Autodesk Fusion 360 part; units mm, degrees
note: some values were not read from the file. Set by a fixed rule: which sketch regions a step uses.
(part 3 of 3)
  line L492 (149.0613, -85.0954) -> (151.4924, -71.3081)
  line L493 (151.4924, -71.3081) -> (165.2797, -73.7391)
  line L494 (165.2797, -73.7391) -> (162.8486, -87.5265)
  line L495 (162.8486, -87.5265) -> (149.0613, -85.0954)
  line L496 (155.3557, -130.0209) -> (152.9246, -143.8082)
  line L497 (152.9246, -143.8082) -> (139.1373, -141.3771)
  line L498 (139.1373, -141.3771) -> (141.5684, -127.5898)
  line L499 (141.5684, -127.5898) -> (155.3557, -130.0209)
  line L500 (139.9031, -107.9523) -> (137.472, -121.7396)
  line L501 (137.472, -121.7396) -> (123.6847, -119.3086)
  line L502 (123.6847, -119.3086) -> (126.1158, -105.5212)
  line L503 (126.1158, -105.5212) -> (139.9031, -107.9523)
  line L504 (158.6637, -111.2603) -> (156.2326, -125.0476)
  line L505 (156.2326, -125.0476) -> (142.4453, -122.6166)
  line L506 (142.4453, -122.6166) -> (144.8764, -108.8292)
  line L507 (144.8764, -108.8292) -> (158.6637, -111.2603)
  line L508 (129.4238, -86.7607) -> (143.2111, -89.1917)
  line L509 (143.2111, -89.1917) -> (140.78, -102.979)
  line L510 (140.78, -102.979) -> (126.9927, -100.548)
  line L511 (126.9927, -100.548) -> (129.4238, -86.7607)
  line L512 (166.1566, -68.7659) -> (152.3693, -66.3348)
  line L513 (152.3693, -66.3348) -> (154.8004, -52.5475)
  line L514 (154.8004, -52.5475) -> (168.5877, -54.9786)
  line L515 (168.5877, -54.9786) -> (166.1566, -68.7659)
  line L516 (107.7824, -70.7088) -> (105.3513, -84.4961)
  line L517 (105.3513, -84.4961) -> (91.564, -82.065)
  line L518 (91.564, -82.065) -> (93.9951, -68.2777)
  line L519 (93.9951, -68.2777) -> (107.7824, -70.7088)
  line L520 (130.2851, -52.7942) -> (127.854, -66.5815)
  line L521 (127.854, -66.5815) -> (114.0667, -64.1504)
  line L522 (114.0667, -64.1504) -> (116.4978, -50.3631)
  line L523 (116.4978, -50.3631) -> (130.2851, -52.7942)
  line L524 (157.0019, -158.2608) -> (176.1466, -49.6857)
  line L525 (176.1466, -49.6857) -> (132.1996, -41.9367)
  arc A0 (56.1359, -6.4676) -> (132.1996, -41.9367) centre (160.3539, 117.7346) ccw
  arc A1 (-132.1996, -41.9367) -> (-56.1359, -6.4676) centre (-160.3539, 117.7346) ccw
  line L526 (-132.1996, -41.9367) -> (-176.1466, -49.6857)
  line L527 (-176.1466, -49.6857) -> (-157.0019, -158.2608)
  line L528 (-157.0019, -158.2608) -> (-24.2252, -134.8487)
  arc A2 (24.2252, -134.8487) -> (-24.2252, -134.8487) centre (0, -272.2365) ccw
  line L529 (24.2252, -134.8487) -> (157.0019, -158.2608)
  line L530 (154.5684, -154.7854) -> (24.7461, -131.8943)
  line L531 (154.5684, -154.7854) -> (172.6712, -52.1192)
  line L532 (172.6712, -52.1192) -> (131.6786, -44.8911)
  line L533 (24.2252, -134.8487) -> (24.7461, -131.8943) construction
  line L534 (132.1996, -41.9367) -> (131.6786, -44.8911) construction
  arc A3 (54.2075, -8.7658) -> (131.6786, -44.8911) centre (160.3539, 117.7346) ccw
  line L535 (0, -2.5) -> (0, -20)
  arc A4 (-131.6786, -44.8911) -> (-54.2075, -8.7658) centre (-160.3539, 117.7346) ccw
  line L536 (-172.6712, -52.1192) -> (-131.6786, -44.8911)
  line L537 (-154.5684, -154.7854) -> (-172.6712, -52.1192)
  line L538 (-154.5684, -154.7854) -> (-24.7461, -131.8943)
  arc A5 (24.7461, -131.8943) -> (-24.7461, -131.8943) centre (0, -272.2365) ccw
  arc A6 (56.1359, -6.4676) -> (38.3662, 0) centre (38.3662, -27.6446) ccw
  line L539 (38.3662, 0) -> (-38.3662, 0)
  arc A7 (-38.3662, 0) -> (-56.1359, -6.4676) centre (-38.3662, -27.6446) ccw
  line L540 (38.3662, -3) -> (-38.3662, -3)
  line L541 (-38.3662, -3) -> (-38.3662, 0) construction
  line L542 (38.3662, -3) -> (38.3662, 0) construction
  arc A8 (54.2075, -8.7658) -> (38.3662, -3) centre (38.3662, -27.6446) ccw
  arc A9 (-38.3662, -3) -> (-54.2075, -8.7658) centre (-38.3662, -27.6446) ccw
  point P0 (54.2075, -8.7658)
  dimension "d428" = 3
  dimension "d429" = 3
  dimension "d430" = 3
  dimension "d431" = 3
  dimension "d436" = 3
  constraint perpendicular L47 L530
  constraint perpendicular L530 L531
  constraint perpendicular L524 L532
  constraint coincident A2.start L529.start
  constraint perpendicular L530 L533
  constraint coincident L525.end A0.end
  constraint perpendicular L532 L534
  constraint coincident L250 P0
  constraint coincident P0 A3.start
  constraint tangent L532 A3
  constraint symmetric L530.start L535 L537.start
  constraint symmetric L530.end L535 L538.end
  constraint symmetric L531.end L535 L536.start
  constraint symmetric L532.end L535 A4.start
  constraint symmetric P0 L535 A4.end
  constraint symmetric A3 L535 A4
  constraint tangent L530 A5
  constraint tangent L538 A5
  constraint horizontal L540
  constraint coincident L539.end A7.start
  constraint coincident A6.end L539.start
  constraint perpendicular L540 L542
  constraint perpendicular L540 L541
  constraint tangent L540 A8
  constraint tangent A4 A9
  measures "d428" distance of L524 L531
  measures "d429" distance of L529 L530
  measures "d430" distance of L525 L532
  measures "d431" distance of A0.start P0
  measures "d436" distance of L539 L540
extrude "Extrusion11" add sketch "Skizze4" along normal up to surface contours L524 L525 A0 A1 L526 L527 L528 A2 L529 A6 L539 A7 end surface through (0, 80, 16.8816) normal (0, 0.043619, -0.999048) offset 0 bodies 1
fillet "Abrundung1" radius 2 12 edges at (166.5742, 103.9733, 0) (154.1731, 45.8112, 0) (91.8329, 29.2091, 0) (47.8213, 1.6672, 0) (0, 0, 0) (-47.8213, 1.6672, 0) (-91.8329, 29.2091, 0) (-154.1731, 45.8112, 0) (-166.5742, 103.9733, 0) (-90.6135, 146.5547, 0) (0, 132.7292, 0) (90.6135, 146.5547, 0) on bodies 1
ref_plane "Arbeitsebene2" through (0, 0, 11) normal (0, 0, 1) x (1, 0, 0)
sketch "Skizze6" plane through (0, 0, 11) normal (0, 0, 1) x (1, 0, 0)
  line L0 (-153.7572, 153.627) -> (-24.9198, 130.9094)
  line L1 (-154.5684, 154.7854) -> (-24.7461, 131.8943)
  line L2 (-24.9198, 130.9094) -> (-24.7461, 131.8943) construction
  line L3 (-153.7572, 153.627) -> (-171.5128, 52.9304)
  line L4 (-172.6712, 52.1192) -> (-154.5684, 154.7854)
  line L5 (-171.5128, 52.9304) -> (-131.505, 45.8759)
  line L6 (-131.6786, 44.8911) -> (-172.6712, 52.1192)
  line L7 (-131.505, 45.8759) -> (-131.6786, 44.8911) construction
  line L8 (-38.3662, 4) -> (38.3662, 4)
  line L9 (38.3662, 3) -> (-38.3662, 3)
  line L10 (38.3662, 3) -> (38.3662, 4) construction
  line L11 (-38.3662, 4) -> (-38.3662, 3) construction
  arc A0 (-53.5647, 9.5318) -> (-131.505, 45.8759) centre (-160.3539, -117.7346) ccw
  arc A1 (-53.5647, 9.5318) -> (-38.3662, 4) centre (-38.3662, 27.6446) ccw
  arc A2 (-54.2075, 8.7658) -> (-131.6786, 44.8911) centre (-160.3539, -117.7346) ccw
  arc A3 (-54.2075, 8.7658) -> (-38.3662, 3) centre (-38.3662, 27.6446) ccw
  line L12 (0, 1.75) -> (0, 22.5)
  arc A4 (38.3662, 4) -> (53.5647, 9.5318) centre (38.3662, 27.6446) ccw
  arc A5 (131.505, 45.8759) -> (53.5647, 9.5318) centre (160.3539, -117.7346) ccw
  line L13 (171.5128, 52.9304) -> (131.505, 45.8759)
  line L14 (153.7572, 153.627) -> (171.5128, 52.9304)
  line L15 (153.7572, 153.627) -> (24.9198, 130.9094)
  arc A6 (-24.9198, 130.9094) -> (24.9198, 130.9094) centre (0, 272.2365) ccw
  line L16 (0, 128.7292) -> (0, 126.7292) construction
  line L17 (0, 126.7292) -> (-11, 126.7292)
  line L18 (-11, 126.7292) -> (-11, 129.1515)
  line L19 (0, 126.7292) -> (11, 126.7292)
  line L20 (11, 126.7292) -> (11, 129.1515)
  dimension "d445" = 1
  dimension "d447" = 1
  dimension "d448" = 1
  dimension "d449" = 1
  dimension "d489" = 2
  dimension "d490" = 11
  dimension "d491" = 11
  constraint parallel L0 L1
  constraint coincident L1.end L2.end
  constraint perpendicular L0 L2
  constraint perpendicular L0 L3
  constraint perpendicular L3 L5
  constraint coincident L6.start L7.end
  constraint perpendicular L5 L7
  constraint parallel L8 L9
  constraint coincident L9.start L10.start
  constraint coincident L9.end L11.end
  constraint perpendicular L8 L11
  constraint perpendicular L8 L10
  constraint tangent L5 A0
  constraint tangent A0 A1
  constraint concentric A0 A2
  constraint concentric A1 A3
  constraint symmetric L0.start L12 L14.start
  constraint symmetric L0.end L12 L15.end
  constraint symmetric L3.end L12 L13.start
  constraint symmetric L5.end L12 A5.start
  constraint symmetric L8.start L12 L8.end
  constraint symmetric A0.start L12 A4.end
  constraint symmetric A0 L12 A5
  constraint symmetric A1 L12 A4
  constraint tangent L0 A6
  constraint tangent L15 A6
  constraint midpoint A6 L16.start
  constraint vertical L16
  constraint perpendicular L16 L17
  constraint coincident A6 L18.end
  constraint perpendicular L17 L18
  constraint perpendicular L16 L19
  constraint coincident A6 L20.end
  constraint perpendicular L19 L20
  measures "d445" distance of L0 L1
  measures "d447" distance of L3 L4
  measures "d448" distance of L5 L6
  measures "d449" distance of L8 L9
  measures "d489" distance of L16.start L16.end
  measures "d490" distance of L16.end L17.end
  measures "d491" distance of L16.end L19.end
extrude "Extrusion12" add sketch "Skizze6" along normal up to surface separate body end surface through (0, 80, 16.8816) normal (0, 0.043619, -0.999048) offset 0 makes body 2
extrude "Extrusion17" add sketch "Skizze6" against normal blind 6 contours A6 L17 L18 L19 L20 bodies 2
ref_plane "Arbeitsebene3" through (0, 78.9443, 13.8327) normal (0, -0.043619, 0.999048) x (1, 0, 0)
sketch "Skizze7" plane through (0, 78.9443, 13.8327) normal (0, -0.043619, 0.999048) x (1, 0, 0)
  line L0 (11, 47.614) -> (-11, 47.614)
  line L1 (0, -77.7242) -> (0, -56.994)
  line L2 (11, 47.614) -> (11, -4.386)
  line L3 (11, -4.386) -> (-11, -4.386)
  line L4 (-11, -4.386) -> (-11, 47.614)
  circle A0 centre (-5.7, -1.886) radius 0.75
  circle A1 centre (5.7, -1.886) radius 0.75
  circle A2 centre (5.7, 45.114) radius 0.75
  circle A3 centre (-5.7, 45.114) radius 0.75
  ellipse E0 centre (0, 192.9846) end of major axis (143.5072, 192.9846) minor radius 143.3707 (-24.9198, 51.7921) -> (-11, 50.0358) ccw
  ellipse E1 centre (0, 192.9846) end of major axis (143.5072, 192.9846) minor radius 143.3707 (11, 50.0358) -> (24.9198, 51.7921) ccw
  point P0 (0, 49.614)
  dimension "d455" = 2
  dimension "d456" = 11
  dimension "d457" = 11
  dimension "d458" = 52
  dimension "d460" = 1.5
  dimension "d461" = 1.5
  dimension "d462" = 2.5
  dimension "d463" = 2.5
  dimension "d464" = 5.3
  dimension "d465" = 5.3
  dimension "d466" = 11.4
  dimension "d467" = 1.5
  dimension "d468" = 1.5
  dimension "d469" = 2.5
  dimension "d470" = 2.5
  dimension "d471" = 5.3
  dimension "d472" = 5.3
  dimension "d473" = 11.4
  constraint horizontal L0
  constraint coincident P0 L1
  constraint perpendicular L0 L2
  constraint perpendicular L2 L3
  constraint perpendicular L0 L4
  measures "d455" distance of L0 P0
  measures "d456" horizontal distance of L0.end P0
  measures "d457" horizontal distance of L0.start P0
  measures "d458" distance of L0.start L2.end
  measures "d460" diameter of A0
  measures "d461" diameter of A1
  measures "d462" distance of L3 A1.centre
  measures "d463" distance of L3 A0.centre
  measures "d464" distance of L4 A0.centre
  measures "d465" distance of L2 A1.centre
  measures "d466" distance of A0.centre A1.centre
  measures "d467" diameter of A2
  measures "d468" diameter of A3
  measures "d469" distance of L0 A3.centre
  measures "d470" distance of L0 A2.centre
  measures "d471" distance of L4 A3.centre
  measures "d472" distance of L2 A2.centre
  measures "d473" distance of A2.centre A3.centre
extrude "Extrusion13" cut sketch "Skizze7" against normal through all contours L0 L2 L3 L4 | A0 | A1 | A2 | A3 bodies 2
extrude "Extrusion14" add sketch "Skizze7" against normal blind 1.5 contours A0 | A1 | A2 | A3 bodies 2
sketch "Skizze8" plane through (0, 126.9656, 5.5434) normal (0, -0.999048, -0.043619) x (1, 0, 0)
  line L0 (-11, 5.4618) -> (11, 5.4618)
  line L1 (11, 5.4618) -> (11, 10.376)
  line L2 (11, 10.376) -> (-11, 10.376)
  line L3 (-11, 10.376) -> (-11, 5.4618)
  line L4 (4.5, 5.376) -> (-4.5, 5.376)
  line L5 (-4.5, 5.376) -> (-4.5, 9.376)
  line L6 (-4.5, 9.376) -> (4.5, 9.376)
  line L7 (4.5, 9.376) -> (4.5, 5.376)
  line L8 (6, 1.376) -> (-6, 1.376)
  line L9 (-6, 1.376) -> (-11, 5.4618) construction
  line L10 (6, 1.376) -> (11, 5.4618) construction
  line L11 (-6, 1.376) -> (-6, 13.376)
  line L12 (6, 1.376) -> (6, 13.376)
  line L13 (6, 13.376) -> (-6, 13.376)
  dimension "d477" = 5
  dimension "d478" = 1
  dimension "d480" = 6.5
  dimension "d482" = 6.5
  dimension "d483" = 9
  dimension "d485" = 9
  dimension "d486" = 12
  dimension "d487" = 12
  constraint horizontal L4
  constraint vertical L5
  constraint horizontal L6
  constraint vertical L7
  constraint horizontal L8
  constraint coincident L0.start L3.end
  constraint coincident L0.end L1.start
  constraint equal L9 L10
  constraint perpendicular L2 L11
  constraint perpendicular L2 L12
  constraint horizontal L13
  measures "d477" distance of L2 L4
  measures "d478" distance of L2 L6
  measures "d480" distance of L1 L7
  measures "d482" distance of L3 L5
  measures "d483" distance of L4.start L4.end
  measures "d485" distance of L2 L8
  measures "d486" distance of L8.start L8.end
  measures "d487" distance of L8 L13
extrude "Extrusion15" cut sketch "Skizze8" against normal through all contours L0 L5 L6 L7 | L0 L4 L5 L7 bodies 2
extrude "Extrusion16" cut sketch "Skizze8" against normal through all contours L0 L2 L5 L6 L7 L11 L12 | L0 L4 L5 L7 L8 L11 L12 | L0 L5 L6 L7 | L0 L4 L5 L7 | L2 L11 L12 L13 bodies 1
equation "Lochabstand = 19.05 mm"
equation "Lochgröße = 14 mm"
equation "Stegbreite = Lochabstand - Lochgröße"
equation "Plattenstärke = 3 mm"
equation "Senkung = Bodendicke / 2"
equation "Wandstärke = 3 mm"
equation "Gehäusehöhe = 17.6 mm + Bodendicke"
equation "Bohrung = 2.5 mm"
equation "Schraubenkopf = 4.5 mm"
equation "Kerbtiefe = 1 mm"
equation "Kerblänge = 5 mm"
equation "Kerbhöhe = 1.5 mm"
equation "Bodendicke = 4 mm"
equation "d2 = Lochgröße"
equation "d3 = Lochgröße"
equation "d6 = Lochgröße"
equation "d7 = Lochgröße"
equation "d9 = Lochgröße"
equation "d10 = Lochgröße"
equation "d11 = Lochgröße"
equation "d12 = Lochgröße"
equation "d13 = Stegbreite"
equation "d14 = Lochgröße"
equation "d15 = Lochgröße"
equation "d16 = Lochgröße"
equation "d17 = Lochgröße"
equation "d128 = Lochgröße"
equation "d129 = Lochgröße"
equation "d130 = Lochgröße"
equation "d131 = Lochgröße"
equation "d132 = Stegbreite"
equation "d133 = Stegbreite"
equation "d134 = Stegbreite"
equation "d135 = Stegbreite"
equation "d136 = Stegbreite"
equation "d137 = Stegbreite"
equation "d138 = Lochgröße"
equation "d139 = Lochgröße"
equation "d140 = Stegbreite"
equation "d142 = Lochgröße"
equation "d143 = Lochgröße"
equation "d144 = Lochgröße"
equation "d145 = Lochgröße"
equation "d146 = Lochgröße"
equation "d147 = Lochgröße"
equation "d148 = Lochgröße"
equation "d149 = Lochgröße"
equation "d150 = Stegbreite"
equation "d151 = Lochgröße"
equation "d152 = Lochgröße"
equation "d153 = Lochgröße"
equation "d154 = Lochgröße"
equation "d155 = Lochgröße"
equation "d156 = Lochgröße"
equation "d157 = Lochgröße"
equation "d158 = Lochgröße"
equation "d159 = Stegbreite"
equation "d160 = Stegbreite"
equation "d161 = Stegbreite"
equation "d162 = Stegbreite"
equation "d163 = Stegbreite"
equation "d164 = Stegbreite"
equation "d165 = Lochgröße"
equation "d166 = Lochgröße"
equation "d167 = Stegbreite"
equation "d169 = Stegbreite"
equation "d170 = Lochgröße"
equation "d171 = Lochgröße"
equation "d172 = Stegbreite"
equation "d176 = Lochgröße"
equation "d177 = Lochgröße"
equation "d180 = Lochgröße"
equation "d181 = Lochgröße"
equation "d191 = Stegbreite"
equation "d201 = Lochgröße"
equation "d202 = Lochgröße"
equation "d203 = Lochgröße"
equation "d204 = Lochgröße"
equation "d205 = Lochgröße"
equation "d206 = Lochgröße"
equation "d207 = Lochgröße"
equation "d208 = Lochgröße"
equation "d209 = Stegbreite"
equation "d210 = Lochgröße"
equation "d211 = Lochgröße"
equation "d212 = Lochgröße"
equation "d213 = Lochgröße"
equation "d214 = Lochgröße"
equation "d215 = Lochgröße"
equation "d218 = Stegbreite"
equation "d219 = Stegbreite"
equation "d220 = Stegbreite"
equation "d221 = Stegbreite"
equation "d222 = Stegbreite"
equation "d224 = Lochgröße"
equation "d225 = Lochgröße"
equation "d226 = Stegbreite"
equation "d227 = Stegbreite"
equation "d232 = Stegbreite"
equation "d258 = 1.5 * Stegbreite + Lochgröße / 2"
equation "d280 = Lochgröße"
equation "d281 = Lochgröße"
equation "d282 = Lochgröße"
equation "d283 = Lochgröße"
equation "d284 = Stegbreite"
equation "d285 = Stegbreite"
equation "d286 = Stegbreite / 2"
equation "d287 = Lochgröße"
equation "d288 = Lochgröße"
equation "d289 = Lochgröße"
equation "d290 = Lochgröße"
equation "d291 = Stegbreite"
equation "d292 = Lochgröße"
equation "d293 = Lochgröße"
equation "d294 = Stegbreite"
equation "d295 = Lochgröße"
equation "d296 = Lochgröße"
equation "d297 = Lochgröße"
equation "d298 = Lochgröße"
equation "d300 = Lochgröße"
equation "d301 = Lochgröße"
equation "d303 = Stegbreite"
equation "d305 = Stegbreite"
equation "d306 = Lochgröße"
equation "d307 = Lochgröße"
equation "d409 = -7 mm + 18.55 mm"
equation "d412 = d409"
equation "d416 = d409"
equation "d420 = d409"
equation "d423 = Stegbreite / 2 + 4 mm"
equation "d424 = d423"
equation "d425 = d423"
equation "d426 = Plattenstärke"
equation "d428 = Wandstärke"
equation "d429 = Wandstärke"
equation "d430 = Wandstärke"
equation "d431 = Wandstärke"
equation "d436 = Wandstärke"
